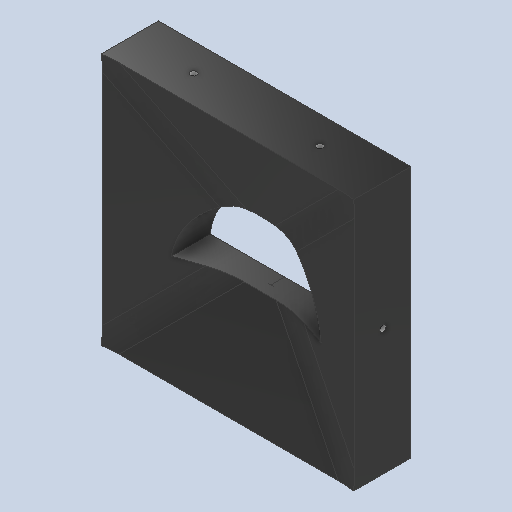
# Autodesk Inventor part: Embudo
Saved by Autodesk Inventor 2023 (Build 270158000, 158)
## iProperties
Created: 2022-12-03
Part Number: Embudo
Material: Genérico
Document SubType Name: Modeling
Designer: sergi
Density: 1 g/cm^3
Appearance: Valor por defecto
Author: sergi
Autodesk Inventor part; units mm, degrees
ref_plane "YZ Plane" through (0, 0, 0) normal (1, 0, 0) x (0, 1, 0)
ref_plane "XZ Plane" through (0, 0, 0) normal (0, 1, 0) x (-1, 0, 0)
ref_plane "XY Plane" through (0, 0, 0) normal (0, 0, 1) x (1, 0, 0)
sketch "Boceto1" plane through (0, 0, 0) normal (0, 0, 1) x (1, 0, 0)
  line L0 (-142.7326, 27.5296) -> (-45.7326, 27.5296) projected
  line L1 (-45.7326, 30.5296) -> (-45.7326, -72.4704) projected
  line L2 (-142.7326, -72.4704) -> (-142.7326, 30.5296) projected
  line L3 (-45.7326, -69.4704) -> (-142.7326, -69.4704) projected
  line L4 (-45.7326, 27.5296) -> (-142.7326, 27.5296)
  line L5 (-142.7326, 27.5296) -> (-142.7326, -69.4704)
  line L6 (-142.7326, -69.4704) -> (-45.7326, -69.4704)
  line L7 (-45.7326, -69.4704) -> (-45.7326, 27.5296)
  dimension "d0" = 97
  dimension "d1" = 97
  constraints: 8 end point, 2 parallel, 1 horizontal, 1 perpendicular
  measures "d0" distance of L6.end L3.end
  measures "d1" distance of L3.end L4.end
extrude "Extrusión1" add sketch "Boceto1" along normal blind 21.5
sketch "Boceto2" plane through (0, 0, 21.5) normal (0, 0, 1) x (1, 0, 0)
  line L0 (-45.7326, -69.4704) -> (-45.7326, 27.5296) projected
  line L1 (-142.7326, 27.5296) -> (-142.7326, -69.4704) projected
  line L2 (-94.2326, -33.4704) -> (-65.2326, -33.4704)
  line L3 (-65.2326, -33.4704) -> (-65.2326, -8.4704)
  line L4 (-65.2326, -8.4704) -> (-94.2326, -8.4704)
  line L5 (-94.2326, -33.4704) -> (-123.2326, -33.4704)
  line L6 (-123.2326, -33.4704) -> (-123.2326, -8.4704)
  line L7 (-123.2326, -8.4704) -> (-94.2326, -8.4704)
  line L8 (-94.2326, -20.9704) -> (-94.2326, -33.4704)
  line L9 (-94.2326, -33.4704) -> (-94.2326, -37.4704)
  arc A0 (-65.5098, -33.4704) -> (-121.2559, -47.9937) centre (-94.2326, -37.4704) ccw
  line L10 (-65.2326, -33.4704) -> (-65.5278, -33.3431)
  line L11 (-110.9419, -13.7681) -> (-123.2326, -8.4704)
  line L12 (-65.2326, -8.4704) -> (-77.5233, -13.7681)
  line L13 (-122.9374, -33.3431) -> (-123.2326, -33.4704)
  line L14 (-45.7326, 27.5296) -> (-83.7093, -10.4471)
  line L15 (-106.7326, -33.4704) -> (-142.7326, -69.4704)
  point P0 (0, 0)
  point P1 (-122.9554, -33.4704)
  dimension "d4" = 29
  dimension "d5" = 25
  dimension "d6" = 29
  dimension "d8" = 4
  constraints: 28 end point, 8 point on circle, 4 point on line, 2 horizontal, 2 parallel, 2 perpendicular, 2 vertical, 1 centre point, 1 coincident
  measures "d4" distance of L4.end L3.end
  measures "d5" distance of L3.end L2.end
  measures "d6" distance of L6.end L7.end
  measures "d8" distance of L2.start L9.end
extrude "Extrusión2" cut sketch "Boceto2" against normal through all contours L5 A0 L2
sketch "Boceto5" plane through (0, 0, 0) normal (0, 0, -1) x (-1, 0, 0)
  arc A0 (122.9554, -33.4704) -> (65.5098, -33.4704) centre (94.2326, -37.4704) ccw projected
  point P0 (0, 0)
  constraints: 1 coincident
hole "Agujero1" at (-94.2326, -37.4704, 0) direction (0, 0, 1) diameter 8 depth 5.2 tip angle 118
ref_plane "Plano de trabajo1" through (0, 0, 5.2) normal (0, 0, -1) x (-1, 0, 0)
sketch "Boceto7" plane through (0, 0, 5.2) normal (0, 0, -1) x (-1, 0, 0)
  line L0 (94.2326, -33.4704) -> (94.2326, -20.9704)
  line L1 (94.2326, -33.4704) -> (106.7326, -33.4704) construction
  point P0 (0, 0)
  dimension "d24" = 90
  constraints: 4 end point, 1 horizontal, 1 perpendicular
  measures "d24" angle of L1 L0
loft "Solevación1" cut section 1 edges at (-45.7326, -20.9704, 21.5) (-94.2326, 27.5296, 21.5) (-142.7326, -20.9704, 21.5) (-94.2326, -69.4704, 21.5) section 2 point at (-94.2326, -20.9704, 5.2)
fillet "Empalme1" radius 20 4 edges at (-64.7209, 8.5413, 15.1184) (-63.7326, -51.4704, 15.4505) (-124.7326, -51.4704, 15.4505) (-123.7442, 8.5413, 15.1184)
sketch "Boceto8" plane through (-142.7326, -69.4704, 0) normal (0, -1, 0) x (1, 0, 0)
  circle A0 centre (72.75, 10.75) radius 1.5 projected
  circle A1 centre (24.25, 10.75) radius 1.5 projected
  circle A2 centre (72.75, 10.75) radius 1.5 projected
  circle A3 centre (90.5, -142) radius 1.25 projected
  circle A4 centre (6.5, -142) radius 1.25 projected
  circle A5 centre (90.5, -64.5) radius 1.5 projected
  circle A6 centre (6.5, -64.5) radius 1.5 projected
  line L0 (30.1283, -58) -> (66.8717, -58) projected
  line L1 (66.8717, -58) -> (66.8717, -76) projected
  line L2 (66.8717, -76) -> (30.1283, -76) projected
  line L3 (30.1283, -76) -> (30.1283, -58) projected
  line L4 (0, -148.5) -> (97, -148.5) projected
  line L5 (97, -148.5) -> (97, 31.5) projected
  line L6 (0, 31.5) -> (97, 31.5) projected
  line L7 (0, -148.5) -> (0, 31.5) projected
  point P0 (142.7326, 0)
hole "Agujero2" at (-118.4826, -69.4704, 10.75) at (-69.9826, -69.4704, 10.75) direction (0, 1, 0) diameter 2.5 depth 5 tip angle 118
sketch "Boceto9" plane through (-142.7326, 27.5296, 0) normal (0, 1, 0) x (1, 0, 0)
  circle A0 centre (72.75, -10.75) radius 1.5 projected
  circle A1 centre (24.25, -10.75) radius 1.5 projected
  point P0 (142.7326, 0)
hole "Agujero3" at (-69.9826, 27.5296, 10.75) at (-118.4826, 27.5296, 10.75) direction (0, -1, 0) diameter 2.5 depth 5 tip angle 118
sketch "Boceto10" plane through (-45.7326, -69.4704, 0) normal (1, 0, 0) x (0, 0, -1)
  circle A0 centre (-10.75, 48.5) radius 1.5 projected
  line L0 (148.5, -3) -> (148.5, 100) projected
  line L1 (148.5, 100) -> (-31.5, 100) projected
  line L2 (-31.5, -3) -> (-31.5, 100) projected
  line L3 (148.5, -3) -> (-31.5, -3) projected
  circle A1 centre (64.5, 90.5) radius 1.5 projected
  circle A2 centre (142, 6.5) radius 1.5 projected
  circle A3 centre (64.5, 6.5) radius 1.5 projected
  circle A4 centre (142, 90.5) radius 1.5 projected
  circle A5 centre (127.92, 10.05) radius 1.5 projected
  circle A6 centre (83.5002, 59.1002) radius 3.0003 projected
  line L4 (9.6, 84.65) -> (34.6, 84.65) projected
  line L5 (34.6, 84.65) -> (34.6, 12.35) projected
  line L6 (34.6, 12.35) -> (9.6, 12.35) projected
  line L7 (9.6, 12.35) -> (9.6, 84.65) projected
  circle A7 centre (6.05, 86.05) radius 1.45 projected
  circle A8 centre (83.5, 71.6001) radius 3.0001 projected
  circle A9 centre (127.92, 39.45) radius 1.5 projected
  circle A10 centre (101.08, 39.45) radius 1.5 projected
  circle A11 centre (83.4996, 37.5996) radius 4.4994 projected
  circle A12 centre (6.05, 11.15) radius 1.45 projected
  circle A13 centre (36.95, 86.05) radius 1.45 projected
  circle A14 centre (36.95, 11.15) radius 1.45 projected
  line L8 (77.6, 16.6) -> (77.6, 27.6) projected
  line L9 (77.6, 27.6) -> (88.6, 27.6) projected
  line L10 (88.6, 27.6) -> (88.6, 16.6) projected
  line L11 (88.6, 16.6) -> (77.6, 16.6) projected
  circle A15 centre (101.08, 10.05) radius 1.5 projected
  point P0 (0, 69.4704)
hole "Agujero4" at (-45.7326, -20.9704, 10.75) direction (-1, 0, 0) diameter 2.5 depth 5 tip angle 118
sketch "Boceto11" plane through (-142.7326, -69.4704, 0) normal (-1, 0, 0) x (0, 0, 1)
  circle A0 centre (10.75, 48.5) radius 1.25 projected
  point P0 (0, 69.4704)
hole "Agujero5" at (-142.7326, -20.9704, 10.75) direction (1, 0, 0) diameter 2.5 depth 5 tip angle 118
